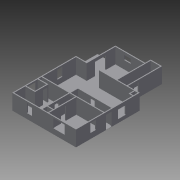
# Autodesk Inventor part: 289 Manning First Floor
Saved by Autodesk Inventor 2013 SP2 (Build 170200200, 200)
## iProperties
Created: 2014-06-09
Part Number: 289 Manning First Floor
Material: Generic
Document SubType Name: Modeling
Designer: jmw3
Density: 1 g/cm^3
Author: jmw3
Autodesk Inventor part; units mm, degrees
ref_plane "YZ Plane" through (0, 0, 0) normal (1, 0, 0) x (0, 1, 0)
ref_plane "XZ Plane" through (0, 0, 0) normal (0, 1, 0) x (-1, 0, 0)
ref_plane "XY Plane" through (0, 0, 0) normal (0, 0, 1) x (1, 0, 0)
sketch "Sketch1" plane through (0, 0, 0) normal (0, 1, 0) x (-1, 0, 0)
  line L0 (-4978.4, 4978.4) -> (4978.4, 4978.4)
  line L1 (4978.4, 4978.4) -> (4978.4, -4978.4)
  line L2 (0, -13370.56) -> (0, 8036.56) projected
  line L3 (8128, 0) -> (-7162.8, 0) projected
  line L4 (-1346.2, -10312.4) -> (-3124.2, -10312.4)
  line L5 (-1346.2, -10312.4) -> (-1346.2, -9448.8)
  line L6 (-1346.2, -9448.8) -> (3302, -9448.8)
  line L7 (3302, -9448.8) -> (3302, -10312.4)
  line L8 (3302, -10312.4) -> (4394.2, -10312.4)
  line L9 (4394.2, -10312.4) -> (4394.2, -9296.4)
  line L10 (4394.2, -9296.4) -> (5943.6, -9296.4)
  line L11 (5943.6, -9296.4) -> (5943.6, -4978.4)
  line L12 (5943.6, -4978.4) -> (3302, -4978.4)
  line L13 (3302, -4978.4) -> (3302, -9448.8)
  line L14 (4978.4, -4978.4) -> (3302, -4978.4)
  line L15 (-3124.2, -4978.4) -> (-4978.4, -4978.4)
  line L16 (4826, 3098.8) -> (4826, 4826)
  line L17 (4826, 4826) -> (558.8, 4826)
  line L18 (558.8, 4826) -> (558.8, 2946.4)
  line L19 (558.8, 2946.4) -> (406.4, 2946.4)
  line L20 (406.4, 4826) -> (-457.2, 4826)
  line L21 (-457.2, 2946.4) -> (-609.6, 2946.4)
  line L22 (-609.6, 2946.4) -> (-609.6, 4826)
  line L23 (-609.6, 4826) -> (-4826, 4826)
  line L24 (-4826, 4826) -> (-4826, 558.8)
  line L25 (-4826, 558.8) -> (-609.6, 558.8)
  line L26 (-609.6, 558.8) -> (-609.6, 2184.4)
  line L27 (-609.6, 2184.4) -> (-457.2, 2184.4)
  line L28 (-457.2, 2184.4) -> (-457.2, 406.4)
  line L29 (-457.2, 406.4) -> (-4826, 406.4)
  line L30 (-4826, 406.4) -> (-4826, 279.4)
  line L31 (-4826, 279.4) -> (-4978.4, 279.4)
  line L32 (4826, 3098.8) -> (3302, 3098.8)
  line L33 (3302, 3098.8) -> (3302, 1854.2)
  line L34 (3302, 1854.2) -> (3454.4, 1854.2)
  line L35 (3454.4, 1854.2) -> (3454.4, 2946.4)
  line L36 (3454.4, 2946.4) -> (4826, 2946.4)
  line L37 (4826, 2946.4) -> (4826, 1168.4)
  line L38 (4826, -4826) -> (3149.6, -4826)
  line L39 (3149.6, -4826) -> (3149.6, -6096)
  line L40 (3149.6, -6096) -> (3302, -6096)
  line L41 (3302, -7823.2) -> (3149.6, -7823.2)
  line L42 (3149.6, -7823.2) -> (3149.6, -9296.4)
  line L43 (3149.6, -9296.4) -> (-1498.6, -9296.4)
  line L44 (-1498.6, -9296.4) -> (-1498.6, -10160)
  line L45 (-1498.6, -10160) -> (-2971.8, -10160)
  line L46 (-2971.8, -10160) -> (-2971.8, -6654.8)
  line L47 (-2971.8, -6654.8) -> (-3124.2, -6654.8)
  line L48 (-3124.2, -5918.2) -> (-2971.8, -5918.2)
  line L49 (-2971.8, -5918.2) -> (-2971.8, -4978.4)
  line L50 (-2971.8, -4978.4) -> (1244.6, -4978.4)
  line L51 (1244.6, -4978.4) -> (1244.6, -4826)
  line L52 (1244.6, -4826) -> (-1117.6, -4826)
  line L53 (-1117.6, -863.6) -> (558.8, -863.6)
  line L54 (558.8, -863.6) -> (558.8, 406.4)
  line L55 (558.8, 406.4) -> (4826, 406.4)
  line L56 (558.8, 2184.4) -> (558.8, 558.8)
  line L57 (558.8, 558.8) -> (4826, 558.8)
  line L58 (558.8, 2184.4) -> (406.4, 2184.4)
  line L59 (406.4, 2184.4) -> (406.4, -711.2)
  line L60 (406.4, -711.2) -> (-1447.8, -711.2)
  line L61 (-1447.8, -711.2) -> (-1447.8, -863.6)
  line L62 (-1447.8, -863.6) -> (-1270, -863.6)
  line L63 (-1270, -4826) -> (-4216.4, -4826)
  line L64 (-4216.4, -4826) -> (-4216.4, -3987.8)
  line L65 (-4216.4, -3987.8) -> (-4826, -3987.8)
  line L66 (-4826, -3987.8) -> (-4826, -863.6)
  line L67 (-4826, -863.6) -> (-2209.8, -863.6)
  line L68 (-2209.8, -863.6) -> (-2209.8, -711.2)
  line L69 (-2209.8, -711.2) -> (-4826, -711.2)
  line L70 (-4826, -711.2) -> (-4826, -584.2)
  line L71 (-4826, -584.2) -> (-4978.4, -584.2)
  line L72 (-4368.8, -4826) -> (-4368.8, -4140.2)
  line L73 (-4368.8, -4140.2) -> (-4826, -4140.2)
  line L74 (-4826, -4140.2) -> (-4826, -4826)
  line L75 (-4826, -4826) -> (-4368.8, -4826)
  line L76 (4826, 1016) -> (4826, 558.8)
  line L77 (4826, 406.4) -> (4826, -4826)
  line L78 (4826, 1168.4) -> (3302, 1168.4)
  line L79 (3302, 1168.4) -> (3302, 1016)
  line L80 (3302, 1016) -> (4826, 1016)
  line L81 (-457.2, 4114.8) -> (406.4, 4114.8)
  line L82 (406.4, 3962.4) -> (-457.2, 3962.4)
  line L83 (-457.2, 4826) -> (-457.2, 4114.8)
  line L84 (-457.2, 3962.4) -> (-457.2, 2946.4)
  line L85 (406.4, 2946.4) -> (406.4, 3962.4)
  line L86 (406.4, 4114.8) -> (406.4, 4826)
  line L87 (-4978.4, -4978.4) -> (-4978.4, -584.2)
  line L88 (-4978.4, 279.4) -> (-4978.4, 4978.4)
  line L89 (-1270, -863.6) -> (-1117.6, -863.6)
  line L90 (-1270, -4826) -> (-1117.6, -4826)
  line L91 (-3124.2, -10312.4) -> (-3124.2, -6654.8)
  line L92 (-3124.2, -5918.2) -> (-3124.2, -4978.4)
  line L93 (-4978.4, 4978.4) -> (4978.4, 4978.4)
  line L94 (4978.4, 4978.4) -> (4978.4, -4978.4)
  line L95 (4978.4, -4978.4) -> (-4978.4, -4978.4)
  line L96 (-4978.4, -4978.4) -> (-4978.4, 4978.4)
  line L97 (-3124.2, -4978.4) -> (3302, -4978.4)
  line L98 (3302, -4978.4) -> (3302, -9448.8)
  line L99 (3302, -9448.8) -> (-3124.2, -9448.8)
  line L100 (-3124.2, -9448.8) -> (-3124.2, -4978.4)
  line L101 (-3124.2, -9448.8) -> (-1346.2, -9448.8)
  line L102 (-1346.2, -9448.8) -> (-1346.2, -10312.4)
  line L103 (-1346.2, -10312.4) -> (-3124.2, -10312.4)
  line L104 (-3124.2, -10312.4) -> (-3124.2, -9448.8)
  line L105 (3302, -4978.4) -> (5943.6, -4978.4)
  line L106 (5943.6, -4978.4) -> (5943.6, -9296.4)
  line L107 (5943.6, -9296.4) -> (3302, -9296.4)
  line L108 (3302, -9296.4) -> (3302, -4978.4)
  line L109 (3302, -9296.4) -> (4394.2, -9296.4)
  line L110 (4394.2, -9296.4) -> (4394.2, -10312.4)
  line L111 (4394.2, -10312.4) -> (3302, -10312.4)
  line L112 (3302, -10312.4) -> (3302, -9296.4)
  point P0 (0, 0)
  dimension "d6" = 863.6
  dimension "d9" = 4648.2
  dimension "d10" = 863.6
  dimension "d11" = 1092.2
  dimension "d12" = 4318
  dimension "d13" = 1549.4
  dimension "d14" = 9956.8
  dimension "d15" = 5334
  dimension "d17" = 152.4
  dimension "d20" = 152.4
  dimension "d21" = 152.4
  dimension "d22" = 152.4
  dimension "d24" = 152.4
  dimension "d25" = 152.4
  dimension "d26" = 152.4
  dimension "d27" = 152.4
  dimension "d28" = 152.4
  dimension "d30" = 152.4
  dimension "d31" = 152.4
  dimension "d32" = 152.4
  dimension "d34" = 152.4
  dimension "d35" = 152.4
  dimension "d37" = 1727.2
  dimension "d38" = 2971.8
  dimension "d45" = 863.6
  dimension "d46" = 1117.6
  dimension "d47" = 152.4
  dimension "d48" = 4419.6
  dimension "d49" = 152.4
  dimension "d50" = 711.2
  dimension "d51" = 152.4
  dimension "d52" = 1879.6
  dimension "d53" = 762
  dimension "d54" = 152.4
  dimension "d55" = 1371.6
  dimension "d56" = 685.8
  dimension "d57" = 990.6
  dimension "d58" = 863.6
  dimension "d59" = 152.4
  dimension "d60" = 9956.8
  dimension "d61" = 2616.2
  dimension "d62" = 762
  dimension "d63" = 4267.2
  dimension "d64" = 609.6
  dimension "d65" = 838.2
  dimension "d66" = 152.4
  dimension "d67" = 3657.6
  dimension "d68" = 736.6
  dimension "d69" = 1854.2
  dimension "d70" = 1778
  dimension "d71" = 1727.2
  dimension "d72" = 1473.2
  dimension "d73" = 1905
  constraints: 222 end point, 61 perpendicular, 59 parallel, 31 collinear, 8 horizontal, 5 point on line, 2 other
  measures "d6" distance between parallel lines of L4 L6
  measures "d9" distance between parallel lines of L7 L5
  measures "d10" distance between parallel lines of L6 L8
  measures "d11" distance from line of L8.end L7
  measures "d12" distance between parallel lines of L12 L10
  measures "d13" distance between parallel lines of L11 L9
  measures "d14" distance between parallel lines of L0 L15
  measures "d15" distance between parallel lines of L15 L4
  measures "d17" distance between parallel lines of L0 L23
  measures "d20" distance between parallel lines of L1 L16
  measures "d21" distance between parallel lines of L36 L32
  measures "d22" distance between parallel lines of L33 L35
  measures "d24" distance between parallel lines of L14 L38
  measures "d25" distance between parallel lines of L13 L39
  measures "d26" distance between parallel lines of L6 L43
  measures "d27" distance between parallel lines of L5 L44
  measures "d28" distance between parallel lines of L4 L45
  measures "d30" distance between parallel lines of L29 L25
  measures "d31" distance between parallel lines of L64 L72
  measures "d32" distance between parallel lines of L65 L73
  measures "d34" distance between parallel lines of L67 L69
  measures "d35" distance between parallel lines of L55 L57
  measures "d37" distance between parallel lines of L17 L32
  measures "d38" distance between parallel lines of L17 L34
  measures "d45" distance between parallel lines of L59 L28
  measures "d46" distance between parallel lines of L60 L29
  measures "d47" distance between parallel lines of L78 L80
  measures "d48" distance between parallel lines of L17 L55
  measures "d49" distance between parallel lines of L82 L81
  measures "d50" distance between parallel lines of L20 L81
  measures "d51" distance between parallel lines of L22 L83
  measures "d52" distance between parallel lines of L21 L23
  measures "d53" distance between parallel lines of L27 L21
  measures "d54" distance between parallel lines of L18 L85
  measures "d55" distance between parallel lines of L37 L35
  measures "d56" distance between parallel lines of L34 L78
  measures "d57" distance between parallel lines of L69 L31
  measures "d58" distance between parallel lines of L31 L71
  measures "d59" distance between parallel lines of L88 L24
  measures "d60" distance between parallel lines of L1 L88
  measures "d61" distance between parallel lines of L66 L68
  measures "d62" distance of L60.end L68.end
  measures "d63" distance between parallel lines of L77 L54
  measures "d64" distance between parallel lines of L74 L64
  measures "d65" distance between parallel lines of L63 L65
  measures "d66" distance between parallel lines of L92 L49
  measures "d67" distance from line of L4 L47.end
  measures "d68" distance of L48.start L47.end
  measures "d69" distance between parallel lines of L87 L92
  measures "d70" distance between parallel lines of L91 L5
  measures "d71" distance between parallel lines of L40 L41
  measures "d72" distance between parallel lines of L43 L41
  measures "d73" distance between parallel lines of L39 L51
extrude "Extrusion1" add sketch "Sketch1" along normal blind 2387.6 contours L0 L2 L20 L83 L81 L82 L84 L21 L22 L23 L24 L25 L26 L27 L28 L29 L30 L31 L88 | L0 L1 L3 L77 L55 L54 L59 L58 L56 L57 L76 L80 L79 L78 L37 L36 L35 L34 L33 L32 L16 L17 L18 L19 L85 L82 L2 L81 L86 L20 | L1 L12 L95 L39 L38 L77 L3 | L71 L70 L69 L68 L67 L66 L65 L64 L63 L90 L52 L2 L50 L95 L15 L87 | L60 L59 L3 L54 L53 L2 | L2 L53 L89 L62 L61 L60 | L13 L40 L39 L95 | L95 L49 L48 L92 | L52 L51 L50 L2 | L13 L6 L2 L43 L42 L41 | L47 L46 L99 L91 | L2 L6 L99 L44 L43 | L99 L46 L45 L44 L5 L4 L91
extrude "Extrusion2" add sketch "Sketch1" against normal blind 25.4 contours L0 L2 L20 L83 L81 L82 L84 L21 L22 L23 L24 L25 L26 L27 L28 L29 L30 L31 L88 | L0 L1 L3 L77 L55 L54 L59 L58 L56 L57 L76 L80 L79 L78 L37 L36 L35 L34 L33 L32 L16 L17 L18 L19 L85 L82 L2 L81 L86 L20 | L31 L30 L29 L28 L27 L26 L25 L24 L23 L22 L21 L84 L82 L2 L3 L96 | L20 L86 L81 L2 | L2 L81 L83 L20 | L3 L2 L60 L61 L62 L89 L53 L52 L90 L63 L64 L65 L66 L67 L68 L69 L70 L71 L96 | L1 L12 L95 L39 L38 L77 L3 | L3 L59 L60 L2 | L2 L82 L85 L19 L18 L17 L16 L32 L33 L34 L35 L36 L37 L78 L79 L80 L76 L57 L56 L58 L59 L3 | L71 L70 L69 L68 L67 L66 L65 L64 L63 L90 L52 L2 L50 L95 L15 L87 | L12 L11 L10 L107 L13 | L77 L38 L39 L95 L51 L52 L2 L53 L54 L3 | L3 L54 L55 L77 | L60 L59 L3 L54 L53 L2 | L2 L53 L89 L62 L61 L60 | L13 L40 L39 L95 | L95 L49 L48 L92 | L13 L41 L42 L43 L2 L50 L95 L39 L40 | L52 L51 L50 L2 | L48 L49 L50 L2 L43 L44 L99 L46 L47 L100 | L9 L8 L7 L13 L107 | L13 L6 L2 L43 L42 L41 | L47 L46 L99 L91 | L2 L6 L99 L44 L43 | L99 L46 L45 L44 L5 L4 L91 | L99 L44 L45 L46 | L75 L74 L73 L72
extrude "Extrusion3" add sketch "Sketch1" against normal blind 25.4 contours L75 L74 L73 L72
sketch "Sketch2" plane through (0, 2387.6, 0) normal (0, 1, 0) x (1, 0, 0)
  line L0 (3124.2, 5918.2) -> (2971.8, 5918.2) projected
  line L1 (3124.2, 5918.2) -> (3124.2, 6654.8) projected
  line L2 (2971.8, 6654.8) -> (3124.2, 6654.8) projected
  line L3 (2971.8, 10160) -> (2971.8, 6654.8) projected
  line L4 (1498.6, 10160) -> (2971.8, 10160) projected
  line L5 (1498.6, 9296.4) -> (1498.6, 10160) projected
  line L6 (-3149.6, 9296.4) -> (1498.6, 9296.4) projected
  line L7 (-3149.6, 7823.2) -> (-3149.6, 9296.4) projected
  line L8 (-3302, 7823.2) -> (-3149.6, 7823.2) projected
  line L9 (-3302, 9448.8) -> (-3302, 7823.2) projected
  line L10 (-3302, 9448.8) -> (-3302, 10312.4) projected
  line L11 (-3302, 10312.4) -> (-4394.2, 10312.4) projected
  line L12 (-4394.2, 10312.4) -> (-4394.2, 9296.4) projected
  line L13 (-4394.2, 9296.4) -> (-5943.6, 9296.4) projected
  line L14 (-5943.6, 9296.4) -> (-5943.6, 4978.4) projected
  line L15 (-5943.6, 4978.4) -> (-4978.4, 4978.4) projected
  line L16 (-3302, 4978.4) -> (-4978.4, 4978.4) projected
  line L17 (-3302, 6096) -> (-3302, 4978.4) projected
  line L18 (-3149.6, 6096) -> (-3302, 6096) projected
  line L19 (-3149.6, 4826) -> (-3149.6, 6096) projected
  line L20 (-4826, 4826) -> (-3149.6, 4826) projected
  line L21 (-4826, -406.4) -> (-4826, 4826) projected
  line L22 (-558.8, -406.4) -> (-4826, -406.4) projected
  line L23 (-558.8, 863.6) -> (-558.8, -406.4) projected
  line L24 (1447.8, 863.6) -> (-558.8, 863.6) projected
  line L25 (1447.8, 711.2) -> (1447.8, 863.6) projected
  line L26 (-406.4, 711.2) -> (1447.8, 711.2) projected
  line L27 (-406.4, -2184.4) -> (-406.4, 711.2) projected
  line L28 (-558.8, -2184.4) -> (-406.4, -2184.4) projected
  line L29 (-558.8, -558.8) -> (-558.8, -2184.4) projected
  line L30 (-4826, -558.8) -> (-558.8, -558.8) projected
  line L31 (-4826, -1016) -> (-4826, -558.8) projected
  line L32 (-3302, -1016) -> (-4826, -1016) projected
  line L33 (-3302, -1168.4) -> (-3302, -1016) projected
  line L34 (-4826, -1168.4) -> (-3302, -1168.4) projected
  line L35 (-4826, -2946.4) -> (-4826, -1168.4) projected
  line L36 (-3454.4, -2946.4) -> (-4826, -2946.4) projected
  line L37 (-3454.4, -1854.2) -> (-3454.4, -2946.4) projected
  line L38 (-3302, -1854.2) -> (-3454.4, -1854.2) projected
  line L39 (-3302, -3098.8) -> (-3302, -1854.2) projected
  line L40 (-4826, -3098.8) -> (-3302, -3098.8) projected
  line L41 (-4826, -4826) -> (-4826, -3098.8) projected
  line L42 (-558.8, -4826) -> (-4826, -4826) projected
  line L43 (-558.8, -2946.4) -> (-558.8, -4826) projected
  line L44 (-406.4, -2946.4) -> (-558.8, -2946.4) projected
  line L45 (-406.4, -3962.4) -> (-406.4, -2946.4) projected
  line L46 (457.2, -3962.4) -> (-406.4, -3962.4) projected
  line L47 (457.2, -2946.4) -> (457.2, -3962.4) projected
  line L48 (609.6, -2946.4) -> (457.2, -2946.4) projected
  line L49 (609.6, -4826) -> (609.6, -2946.4) projected
  line L50 (4826, -4826) -> (609.6, -4826) projected
  line L51 (4826, -558.8) -> (4826, -4826) projected
  line L52 (609.6, -558.8) -> (4826, -558.8) projected
  line L53 (609.6, -2184.4) -> (609.6, -558.8) projected
  line L54 (457.2, -2184.4) -> (609.6, -2184.4) projected
  line L55 (457.2, -406.4) -> (457.2, -2184.4) projected
  line L56 (4826, -406.4) -> (457.2, -406.4) projected
  line L57 (4826, -279.4) -> (4826, -406.4) projected
  line L58 (4978.4, -279.4) -> (4826, -279.4) projected
  line L59 (4978.4, -279.4) -> (4978.4, 584.2) projected
  line L60 (4826, 584.2) -> (4978.4, 584.2) projected
  line L61 (4826, 711.2) -> (4826, 584.2) projected
  line L62 (2209.8, 711.2) -> (4826, 711.2) projected
  line L63 (2209.8, 863.6) -> (2209.8, 711.2) projected
  line L64 (4826, 863.6) -> (2209.8, 863.6) projected
  line L65 (4826, 3987.8) -> (4826, 863.6) projected
  line L66 (4216.4, 3987.8) -> (4826, 3987.8) projected
  line L67 (4216.4, 4826) -> (4216.4, 3987.8) projected
  line L68 (-1244.6, 4826) -> (4216.4, 4826) projected
  line L69 (-1244.6, 4978.4) -> (-1244.6, 4826) projected
  line L70 (2971.8, 4978.4) -> (-1244.6, 4978.4) projected
  line L71 (2971.8, 5918.2) -> (2971.8, 4978.4) projected
  line L72 (4368.8, 4140.2) -> (4368.8, 4826) projected
  line L73 (4826, 4140.2) -> (4368.8, 4140.2) projected
  line L74 (4826, 4826) -> (4826, 4140.2) projected
  line L75 (4368.8, 4826) -> (4826, 4826) projected
  line L76 (4978.4, 584.2) -> (4978.4, 4978.4) projected
  line L77 (4978.4, 4978.4) -> (3124.2, 4978.4) projected
  line L78 (3124.2, 6654.8) -> (3124.2, 10312.4) projected
  line L79 (3124.2, 4978.4) -> (3124.2, 5918.2) projected
  line L80 (3124.2, 10312.4) -> (1346.2, 10312.4) projected
  line L81 (1346.2, 9448.8) -> (-3302, 9448.8) projected
  line L82 (-3302, 7823.2) -> (-3149.6, 7823.2) projected
  line L83 (-3149.6, 7823.2) -> (-3149.6, 9296.4) projected
  line L84 (-3149.6, 9296.4) -> (1498.6, 9296.4) projected
  line L85 (1498.6, 9296.4) -> (1498.6, 10160) projected
  line L86 (1498.6, 10160) -> (2971.8, 10160) projected
  line L87 (2971.8, 10160) -> (2971.8, 6654.8) projected
  line L88 (2971.8, 6654.8) -> (3124.2, 6654.8) projected
  line L89 (3124.2, 6654.8) -> (3124.2, 10312.4) projected
  line L90 (3124.2, 10312.4) -> (1346.2, 10312.4) projected
  line L91 (1346.2, 10312.4) -> (1346.2, 9448.8) projected
  line L92 (1346.2, 9448.8) -> (-3302, 9448.8) projected
  line L93 (-3302, 9448.8) -> (-3302, 7823.2) projected
  line L94 (-3302, 7823.2) -> (-3149.6, 7823.2)
  line L95 (-3149.6, 7823.2) -> (-3149.6, 6096)
  line L96 (-3149.6, 6096) -> (-3302, 6096)
  line L97 (-3302, 6096) -> (-3302, 7823.2)
  line L98 (2971.8, 6654.8) -> (3124.2, 6654.8)
  line L99 (3124.2, 6654.8) -> (3124.2, 5918.2)
  line L100 (3124.2, 5918.2) -> (2971.8, 5918.2)
  line L101 (2971.8, 5918.2) -> (2971.8, 6654.8)
  line L102 (1447.8, 863.6) -> (2209.8, 863.6)
  line L103 (2209.8, 863.6) -> (2209.8, 711.2)
  line L104 (2209.8, 711.2) -> (1447.8, 711.2)
  line L105 (1447.8, 711.2) -> (1447.8, 863.6)
  line L106 (-558.8, -2184.4) -> (-406.4, -2184.4)
  line L107 (-406.4, -2184.4) -> (-406.4, -2946.4)
  line L108 (-406.4, -2946.4) -> (-558.8, -2946.4)
  line L109 (-558.8, -2946.4) -> (-558.8, -2184.4)
  line L110 (457.2, -2184.4) -> (609.6, -2184.4)
  line L111 (609.6, -2184.4) -> (609.6, -2946.4)
  line L112 (609.6, -2946.4) -> (457.2, -2946.4)
  line L113 (457.2, -2946.4) -> (457.2, -2184.4)
  line L114 (4826, 584.2) -> (4978.4, 584.2)
  line L115 (4978.4, 584.2) -> (4978.4, -279.4)
  line L116 (4978.4, -279.4) -> (4826, -279.4)
  line L117 (4826, -279.4) -> (4826, 584.2)
  line L118 (-3454.4, -1168.4) -> (-3302, -1168.4)
  line L119 (-3302, -1168.4) -> (-3302, -1854.2)
  line L120 (-3302, -1854.2) -> (-3454.4, -1854.2)
  line L121 (-3454.4, -1854.2) -> (-3454.4, -1168.4)
  line L122 (457.2, -406.4) -> (-406.4, -406.4)
  line L123 (-406.4, -406.4) -> (-406.4, -558.8)
  line L124 (-406.4, -558.8) -> (457.2, -558.8)
  line L125 (457.2, -558.8) -> (457.2, -406.4)
  line L126 (-3149.6, 7823.2) -> (-3302, 7823.2)
  line L127 (-3302, 7823.2) -> (-3302, 6096)
  line L128 (-3302, 6096) -> (-3149.6, 6096)
  line L129 (-3149.6, 6096) -> (-3149.6, 7823.2)
  line L130 (-3149.6, 9296.4) -> (-3149.6, 4826)
  line L131 (-3149.6, 7823.2) -> (-3302, 7823.2)
  line L132 (-3302, 7823.2) -> (-3302, 6096)
  line L133 (-3302, 6096) -> (-3149.6, 6096)
  point P0 (0, 0)
  constraints: 80 end point, 18 parallel, 11 perpendicular, 9 horizontal, 2 collinear, 2 point on line
extrude "Extrusion4" add sketch "Sketch2" against normal blind 457.2 contours L8 L95 L18 L97
extrude "Extrusion5" add sketch "Sketch2" against normal blind 355.6 contours L0 L101 L2 L1 | L59 L58 L117 L60 | L104 L25 L102 L63 | L55 L124 L27 L122 | L54 L111 L48 L113 | L107 L44 L109 L28 | L119 L38 L121 L34
sketch "Sketch3" plane through (-4978.4, 2387.6, 4978.4) normal (0, 0, 1) x (1, 0, 0)
  line L0 (9956.8, -2413) -> (9956.8, 0) projected
  line L1 (0, 0) -> (9956.8, 0) projected
  line L2 (0, -2413) -> (0, 0) projected
  line L3 (9956.8, -2413) -> (0, -2413) projected
  line L4 (4419.6, -2387.6) -> (152.4, -2387.6) projected
  line L5 (9804.4, -2387.6) -> (5588, -2387.6) projected
  line L6 (6426.2, -228.6) -> (8204.2, -228.6)
  line L7 (8204.2, -228.6) -> (8204.2, -1600.2)
  line L8 (8204.2, -1600.2) -> (6426.2, -1600.2)
  line L9 (6426.2, -1600.2) -> (6426.2, -228.6)
  line L10 (2286, -228.6) -> (3073.4, -228.6)
  line L11 (3073.4, -228.6) -> (3073.4, -1600.2)
  line L12 (3073.4, -1600.2) -> (2286, -1600.2)
  line L13 (2286, -1600.2) -> (2286, -228.6)
  point P0 (4978.4, -2387.6)
  dimension "d84" = 2286
  dimension "d85" = 787.4
  dimension "d86" = 787.4
  dimension "d87" = 228.6
  dimension "d88" = 1752.6
  dimension "d89" = 1778
  dimension "d90" = 787.4
  dimension "d91" = 228.6
  constraints: 16 end point, 4 parallel, 2 horizontal, 2 perpendicular
  measures "d84" distance between parallel lines of L2 L13
  measures "d85" distance between parallel lines of L11 L13
  measures "d86" distance between parallel lines of L4 L12
  measures "d87" distance between parallel lines of L1 L10
  measures "d88" distance between parallel lines of L7 L0
  measures "d89" distance between parallel lines of L7 L9
  measures "d90" distance between parallel lines of L5 L8
  measures "d91" distance between parallel lines of L1 L6
extrude "Extrusion6" cut sketch "Sketch3" against normal up to surface (152.4 mm away) contours L6 L7 L8 L9 | L10 L11 L12 L13
sketch "Sketch4" plane through (4978.4, 2387.6, 4978.4) normal (1, 0, 0) x (0, 0, -1)
  line L0 (0, 0) -> (9956.8, 0) projected
  line L1 (0, -2413) -> (0, 0) projected
  line L2 (9956.8, 0) -> (9956.8, -2413) projected
  line L3 (2260.6, -228.6) -> (3124.2, -228.6)
  line L4 (3124.2, -228.6) -> (3124.2, -1600.2)
  line L5 (3124.2, -1600.2) -> (2260.6, -1600.2)
  line L6 (2260.6, -1600.2) -> (2260.6, -228.6)
  line L7 (4419.6, -2387.6) -> (152.4, -2387.6) projected
  line L8 (8966.2, -2387.6) -> (5842, -2387.6) projected
  line L9 (6578.6, -584.2) -> (7772.4, -584.2)
  line L10 (7772.4, -584.2) -> (7772.4, -1879.6)
  line L11 (7772.4, -1879.6) -> (6578.6, -1879.6)
  line L12 (6578.6, -1879.6) -> (6578.6, -584.2)
  point P0 (4978.4, -2387.6)
  dimension "d94" = 2260.6
  dimension "d95" = 863.6
  dimension "d96" = 787.4
  dimension "d97" = 228.6
  dimension "d98" = 2184.4
  dimension "d99" = 1193.8
  dimension "d100" = 584.2
  dimension "d101" = 508
  constraints: 16 end point, 4 parallel, 2 horizontal, 2 perpendicular
  measures "d94" distance between parallel lines of L1 L6
  measures "d95" distance between parallel lines of L4 L6
  measures "d96" distance between parallel lines of L7 L5
  measures "d97" distance between parallel lines of L0 L3
  measures "d98" distance between parallel lines of L2 L10
  measures "d99" distance between parallel lines of L10 L12
  measures "d100" distance between parallel lines of L0 L9
  measures "d101" distance between parallel lines of L8 L11
extrude "Extrusion7" cut sketch "Sketch4" against normal up to surface (152.4 mm away)
sketch "Sketch5" plane through (-3149.6, 2387.6, -9296.4) normal (0, 0, 1) x (1, 0, 0)
  line L0 (0, -2387.6) -> (4648.2, -2387.6) projected
  line L1 (0, 0) -> (4648.2, 0) projected
  line L2 (-152.4, -2387.6) -> (-152.4, 0) projected
  line L3 (4495.8, 0) -> (-152.4, 0) projected
  line L4 (4495.8, -2413) -> (4495.8, 0) projected
  line L5 (-152.4, -2413) -> (4495.8, -2413) projected
  line L6 (-152.4, -2387.6) -> (-152.4, -2413) projected
  line L7 (1346.2, -431.8) -> (2387.6, -431.8)
  line L8 (2387.6, -431.8) -> (2387.6, -1117.6)
  line L9 (2387.6, -1117.6) -> (1346.2, -1117.6)
  line L10 (1346.2, -1117.6) -> (1346.2, -431.8)
  point P0 (3149.6, -2387.6)
  dimension "d104" = 1041.4
  dimension "d106" = 1498.6
  dimension "d107" = 1270
  dimension "d108" = 431.8
  constraints: 8 end point, 2 parallel, 1 horizontal, 1 perpendicular
  measures "d104" distance between parallel lines of L10 L8
  measures "d106" distance between parallel lines of L2 L10
  measures "d107" distance between parallel lines of L0 L9
  measures "d108" distance between parallel lines of L1 L7
extrude "Extrusion8" cut sketch "Sketch5" against normal up to surface (152.4 mm away) contours L7 L8 L9 L10
sketch "Sketch6" plane through (-4978.4, 2387.6, -4978.4) normal (-1, 0, 0) x (0, 0, 1)
  line L0 (9956.8, -2413) -> (9956.8, 0) projected
  line L1 (0, 0) -> (9956.8, 0) projected
  line L2 (5384.8, -2387.6) -> (152.4, -2387.6) projected
  line L3 (7924.8, -2387.6) -> (6146.8, -2387.6) projected
  line L4 (9804.4, -2387.6) -> (8077.2, -2387.6) projected
  line L5 (2286, -228.6) -> (3073.4, -228.6)
  line L6 (3073.4, -228.6) -> (3073.4, -1600.2)
  line L7 (3073.4, -1600.2) -> (2286, -1600.2)
  line L8 (2286, -1600.2) -> (2286, -228.6)
  line L9 (6426.2, -228.6) -> (7924.8, -228.6)
  line L10 (7924.8, -228.6) -> (7924.8, -1600.2)
  line L11 (7924.8, -1600.2) -> (6426.2, -1600.2)
  line L12 (6426.2, -1600.2) -> (6426.2, -228.6)
  point P0 (4978.4, -2387.6)
  dimension "d111" = 6883.4
  dimension "d112" = 787.4
  dimension "d113" = 787.4
  dimension "d114" = 228.6
  dimension "d115" = 787.4
  dimension "d116" = 228.6
  dimension "d117" = 1498.6
  dimension "d118" = 2032
  constraints: 16 end point, 4 parallel, 2 horizontal, 2 perpendicular
  measures "d111" distance between parallel lines of L0 L6
  measures "d112" distance between parallel lines of L8 L6
  measures "d113" distance between parallel lines of L2 L7
  measures "d114" distance between parallel lines of L1 L5
  measures "d115" distance between parallel lines of L3 L11
  measures "d116" distance between parallel lines of L1 L9
  measures "d117" distance between parallel lines of L12 L10
  measures "d118" distance between parallel lines of L0 L10
extrude "Extrusion9" cut sketch "Sketch6" against normal up to surface (152.4 mm away)
sketch "Sketch7" plane through (0, 0, 0) normal (0, 1, 0) x (1, 0, 0)
  line L0 (-3149.6, 9296.4) -> (1498.6, 9296.4) projected
  line L1 (2971.8, 4978.4) -> (-1244.6, 4978.4) projected
  line L2 (3124.2, 10312.4) -> (3124.2, 4978.4) projected
  line L3 (3124.2, 4978.4) -> (4978.4, 4978.4) projected
  line L4 (4978.4, 4978.4) -> (4978.4, -4978.4) projected
  line L5 (4978.4, -4978.4) -> (-4978.4, -4978.4) projected
  line L6 (-4978.4, -4978.4) -> (-4978.4, 4978.4) projected
  line L7 (-4978.4, 4978.4) -> (-5943.6, 4978.4) projected
  line L8 (-5943.6, 4978.4) -> (-5943.6, 9296.4) projected
  line L9 (-5943.6, 9296.4) -> (-4394.2, 9296.4) projected
  line L10 (-4394.2, 9296.4) -> (-4394.2, 10312.4) projected
  line L11 (-4394.2, 10312.4) -> (-3302, 10312.4) projected
  line L12 (-3302, 10312.4) -> (-3302, 9448.8) projected
  line L13 (-3302, 9448.8) -> (1346.2, 9448.8) projected
  line L14 (1346.2, 9448.8) -> (1346.2, 10312.4) projected
  line L15 (1346.2, 10312.4) -> (3124.2, 10312.4) projected
  line L16 (1346.2, 9296.4) -> (1498.6, 9296.4)
  line L17 (1498.6, 9296.4) -> (1498.6, 4978.4)
  line L18 (1498.6, 4978.4) -> (1346.2, 4978.4)
  line L19 (1346.2, 4978.4) -> (1346.2, 9296.4)
  line L20 (3124.2, 5918.2) -> (2971.8, 5918.2) projected
  line L21 (3124.2, 5918.2) -> (3124.2, 6654.8) projected
  line L22 (2971.8, 6654.8) -> (3124.2, 6654.8) projected
  line L23 (2971.8, 10160) -> (2971.8, 6654.8) projected
  line L24 (1498.6, 10160) -> (2971.8, 10160) projected
  line L25 (1498.6, 9296.4) -> (1498.6, 10160) projected
  line L26 (-3149.6, 9296.4) -> (1498.6, 9296.4) projected
  line L27 (-3149.6, 7823.2) -> (-3149.6, 9296.4) projected
  line L28 (-3302, 7823.2) -> (-3149.6, 7823.2) projected
  line L29 (-3302, 9448.8) -> (-3302, 7823.2) projected
  line L30 (-3302, 9448.8) -> (-3302, 10312.4) projected
  line L31 (-3302, 10312.4) -> (-4394.2, 10312.4) projected
  line L32 (-4394.2, 10312.4) -> (-4394.2, 9296.4) projected
  line L33 (-4394.2, 9296.4) -> (-5943.6, 9296.4) projected
  line L34 (-5943.6, 9296.4) -> (-5943.6, 4978.4) projected
  line L35 (-5943.6, 4978.4) -> (-4978.4, 4978.4) projected
  line L36 (-3302, 4978.4) -> (-4978.4, 4978.4) projected
  line L37 (-3302, 6096) -> (-3302, 4978.4) projected
  line L38 (-3149.6, 6096) -> (-3302, 6096) projected
  line L39 (-3149.6, 4826) -> (-3149.6, 6096) projected
  line L40 (-4826, 4826) -> (-3149.6, 4826) projected
  line L41 (-4826, -406.4) -> (-4826, 4826) projected
  line L42 (-558.8, -406.4) -> (-4826, -406.4) projected
  line L43 (-558.8, 863.6) -> (-558.8, -406.4) projected
  line L44 (1447.8, 863.6) -> (-558.8, 863.6) projected
  line L45 (1447.8, 711.2) -> (1447.8, 863.6) projected
  line L46 (-406.4, 711.2) -> (1447.8, 711.2) projected
  line L47 (-406.4, -2184.4) -> (-406.4, 711.2) projected
  line L48 (-558.8, -2184.4) -> (-406.4, -2184.4) projected
  line L49 (-558.8, -558.8) -> (-558.8, -2184.4) projected
  line L50 (-4826, -558.8) -> (-558.8, -558.8) projected
  line L51 (-4826, -1016) -> (-4826, -558.8) projected
  line L52 (-3302, -1016) -> (-4826, -1016) projected
  line L53 (-3302, -1168.4) -> (-3302, -1016) projected
  line L54 (-4826, -1168.4) -> (-3302, -1168.4) projected
  line L55 (-4826, -2946.4) -> (-4826, -1168.4) projected
  line L56 (-3454.4, -2946.4) -> (-4826, -2946.4) projected
  line L57 (-3454.4, -1854.2) -> (-3454.4, -2946.4) projected
  line L58 (-3302, -1854.2) -> (-3454.4, -1854.2) projected
  line L59 (-3302, -3098.8) -> (-3302, -1854.2) projected
  line L60 (-4826, -3098.8) -> (-3302, -3098.8) projected
  line L61 (-4826, -4826) -> (-4826, -3098.8) projected
  line L62 (-558.8, -4826) -> (-4826, -4826) projected
  line L63 (-558.8, -2946.4) -> (-558.8, -4826) projected
  line L64 (-406.4, -2946.4) -> (-558.8, -2946.4) projected
  line L65 (-406.4, -3962.4) -> (-406.4, -2946.4) projected
  line L66 (457.2, -3962.4) -> (-406.4, -3962.4) projected
  line L67 (457.2, -2946.4) -> (457.2, -3962.4) projected
  line L68 (609.6, -2946.4) -> (457.2, -2946.4) projected
  line L69 (609.6, -4826) -> (609.6, -2946.4) projected
  line L70 (4826, -4826) -> (609.6, -4826) projected
  line L71 (4826, -558.8) -> (4826, -4826) projected
  line L72 (609.6, -558.8) -> (4826, -558.8) projected
  line L73 (609.6, -2184.4) -> (609.6, -558.8) projected
  line L74 (457.2, -2184.4) -> (609.6, -2184.4) projected
  line L75 (457.2, -406.4) -> (457.2, -2184.4) projected
  line L76 (4826, -406.4) -> (457.2, -406.4) projected
  line L77 (4826, -279.4) -> (4826, -406.4) projected
  line L78 (4978.4, -279.4) -> (4826, -279.4) projected
  line L79 (4978.4, -279.4) -> (4978.4, 584.2) projected
  line L80 (4826, 584.2) -> (4978.4, 584.2) projected
  line L81 (4826, 711.2) -> (4826, 584.2) projected
  line L82 (2209.8, 711.2) -> (4826, 711.2) projected
  line L83 (2209.8, 863.6) -> (2209.8, 711.2) projected
  line L84 (4826, 863.6) -> (2209.8, 863.6) projected
  line L85 (4826, 3987.8) -> (4826, 863.6) projected
  line L86 (4216.4, 3987.8) -> (4826, 3987.8) projected
  line L87 (4216.4, 4826) -> (4216.4, 3987.8) projected
  line L88 (-1244.6, 4826) -> (4216.4, 4826) projected
  line L89 (-1244.6, 4978.4) -> (-1244.6, 4826) projected
  line L90 (2971.8, 4978.4) -> (-1244.6, 4978.4) projected
  line L91 (2971.8, 5918.2) -> (2971.8, 4978.4) projected
  line L92 (1498.6, 9296.4) -> (1498.6, 10160) projected
  line L93 (1346.2, 10312.4) -> (1346.2, 9448.8) projected
  point P0 (0, 0)
  constraints: 8 end point, 2 collinear, 2 parallel, 2 point on line, 1 horizontal, 1 perpendicular
extrude "Extrusion10" add sketch "Sketch7" along normal up to surface (2387.6 mm away) contours L0 L17 L1 L19
body "Solid1"
